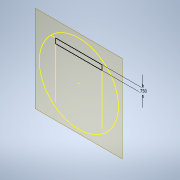
# Autodesk Inventor part: frontSupportFor12inchBase
Saved by Autodesk Inventor 2021 (Build 250183000, 183)
## iProperties
Created: 2020-07-01
Part Number: frontSupportFor12inchBase
Material: Generic
Document SubType Name: Modeling
Designer: robst
Density: 1 g/cm^3
Appearance: Default
Author: robst
Autodesk Inventor part; units mm, degrees
ref_plane "YZ Plane" through (0, 0, 0) normal (1, 0, 0) x (0, 1, 0)
ref_plane "XZ Plane" through (0, 0, 0) normal (0, 1, 0) x (-1, 0, 0)
ref_plane "XY Plane" through (0, 0, 0) normal (0, 0, 1) x (1, 0, 0)
ref_plane "Work Plane1" through (0, 0, 0) normal (0, 0, 1) x (1, 0, 0)
sketch "Sketch1" plane through (0, 0, 0) normal (0, 0, 1) x (1, 0, 0)
  circle A0 centre (0, 0) radius 152.4 projected
  line L0 (88.9, 107.5758) -> (88.9, -107.5758) projected
  line L1 (-88.9, 107.5758) -> (-88.9, -107.5758) projected
  line L2 (-107.95, 107.5758) -> (-88.9, 107.5758) projected
  line L3 (107.95, 107.5758) -> (88.9, 107.5758) projected
  line L4 (88.9, 107.5758) -> (-88.9, 107.5758)
  line L5 (-88.9, 107.5758) -> (-88.9, 88.5258)
  line L6 (-88.9, 88.5258) -> (88.9, 88.5258)
  line L7 (88.9, 88.5258) -> (88.9, 107.5758)
  dimension "d0" = 19.05
  constraints: 8 end point, 2 point on line, 1 collinear, 1 horizontal, 1 perpendicular
  measures "d0" distance between parallel lines of L6 L4
extrude "Extrusion1" add sketch "Sketch1" along normal blind 101.6 contours L0 L6 L1 L4
body "Solid1"
